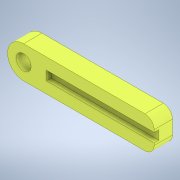
# Autodesk Inventor part: espcam-mount
Saved by Autodesk Inventor 2020 (Build 240168000, 168)
## iProperties
Created: 2020-11-05
Part Number: espcam-mount
Material: Generic
Document SubType Name: Modeling
Designer: alnwlsn
Density: 1 g/cm^3
Appearance: Default
Author: alnwlsn
Autodesk Inventor part; units mm, degrees
ref_plane "YZ Plane" through (0, 0, 0) normal (1, 0, 0) x (0, 1, 0)
ref_plane "XZ Plane" through (0, 0, 0) normal (0, 1, 0) x (-1, 0, 0)
ref_plane "XY Plane" through (0, 0, 0) normal (0, 0, 1) x (1, 0, 0)
sketch "Sketch1" plane through (0, 0, 0) normal (0, 0, 1) x (1, 0, 0)
  circle A0 centre (0, 0) radius 1.65
  arc A1 (0, 3.5) -> (0, -3.5) centre (0, 0) ccw
  line L0 (0, 3.5) -> (26.5, 3.5)
  line L1 (28.5, 1.5) -> (28.5, -1.5)
  line L2 (26.5, -3.5) -> (0, -3.5)
  arc A2 (28.5, 1.5) -> (26.5, 3.5) centre (26.5, 1.5) ccw
  arc A3 (26.5, -3.5) -> (28.5, -1.5) centre (26.5, -1.5) ccw
  dimension "d0" = 3.3
  dimension "d1" = 7
  dimension "d2" = 2
  dimension "d3" = 28.5
  constraints: 6 end point, 6 point on circle, 6 tangent, 4 centre point, 2 coincident, 2 horizontal, 1 equal radius, 1 perpendicular
  measures "d0" diameter of A0
  measures "d1" diameter of A1
  measures "d2" radius of A2
  measures "d3" distance from line of L1 point (0, 0)
extrude "Extrusion1" add sketch "Sketch1" along normal blind 4
sketch "Sketch2" plane through (0, 0, 4) normal (0, 0, 1) x (1, 0, 0)
  line L0 (52, -1) -> (5, -1)
  line L1 (5, -1) -> (5, 1)
  line L2 (5, 1) -> (52, 1)
  line L3 (52, 1) -> (52, -1)
  line L4 (28.5, -1.5) -> (28.5, 1.5) projected
  line L5 (52, -1) -> (5, 1) construction
  line L6 (5, -1) -> (52, 1) construction
  point P0 (0, 0)
  point P1 (28.5, 0)
  point P2 (28.5, -1)
  point P3 (28.5, 1)
  dimension "d6" = 2
  dimension "d7" = 5
  constraints: 12 end point, 3 midpoint, 2 parallel, 1 horizontal, 1 perpendicular
  measures "d6" distance of L0.end L1.end
  measures "d7" distance from line of L1 point (0, 0)
extrude "Extrusion2" cut sketch "Sketch2" against normal blind 1 contours L0 L1 L2 L4
body "Solid1"
